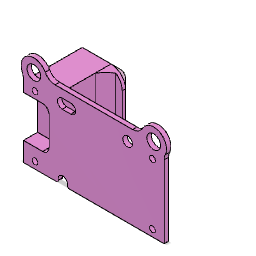
Vindriktning-Cubecell-Mount (Autodesk Fusion 360 design; units mm, degrees)
Autodesk Fusion 360 part; units mm, degrees
sketch "Sketch1" plane through (0, 0, 0) normal (0, 0, 1) x (1, 0, 0)
  line L0 (18.75, 13) -> (-18.75, 13)
  line L1 (-18.75, 13) -> (-18.75, -13)
  line L2 (-18.75, -13) -> (18.75, -13)
  line L3 (18.75, -13) -> (18.75, 13)
  line L4 (18.75, 13) -> (-18.75, -13) construction
  line L5 (-18.75, 13) -> (18.75, -13) construction
  circle A0 centre (18.75, 13) radius 2
  circle A1 centre (-18.75, 13) radius 2
  circle A2 centre (-18.75, 13) radius 4
  circle A3 centre (18.75, 13) radius 4
  line L6 (-18.75, 13) -> (-22, 13)
  line L7 (-22, 13) -> (-22, -13)
  line L8 (-22, -13) -> (-18.75, -13)
  line L9 (-18.75, -13) -> (-18.75, 13)
  line L10 (0, 6) -> (0, -5)
  line L11 (18.75, -13) -> (18.75, 13)
  line L12 (18.75, 13) -> (22, 13)
  line L13 (22, -13) -> (18.75, -13)
  line L14 (22, 13) -> (22, -13)
  line L15 (-22, -6) -> (-14, -6)
  line L16 (-14, -6) -> (-14, 6)
  line L17 (-14, 6) -> (-22, 6)
  line L18 (-22, 6) -> (-22, -6)
  circle A4 centre (-18.75, 13) radius 2.15
  circle A5 centre (18.75, 13) radius 2.15
  dimension "d1" = 37.5
  dimension "d2" = 26
  dimension "d3" = 4
  dimension "d4" = 4
  dimension "d5" = 2
  dimension "d6" = 2
  dimension "d7" = 8
  dimension "d8" = 0.15
  dimension "d9" = 0.15
  constraint horizontal L0
  constraint perpendicular L0 L1
  constraint parallel L0 L2
  constraint parallel L1 L3
  constraint coincident L4 origin
  constraint coincident L5 origin
  constraint coincident L0.start L3.end
  constraint coincident L0.end L1.start
  constraint horizontal L6
  constraint vertical L7
  constraint horizontal L8
  constraint vertical L9
  constraint vertical L10
  constraint symmetric L0.end L10 L0.start
  constraint symmetric L6.end L10 L12.end
  constraint symmetric L7.end L10 L13.start
  constraint symmetric L1.end L10 L2.end
  constraint horizontal L15
  constraint vertical L16
  constraint horizontal L17
  constraint vertical L18
  constraint coincident L7 L15.start
  measures "d1" distance of L1.end L2.end
  measures "d2" distance of L0.end L1.end
  measures "d3" diameter of A0
  measures "d4" diameter of A1
  measures "d5" distance of A1
  measures "d6" distance of A0
  measures "d7" distance of L15.start L15.end
extrude "Extrude1" add sketch "Sketch1" along normal blind 1.4 contours L0 L1 A2 L9 A4 | L0 A2 L6 L7 A4 | L0 L1 L2 L3 A2 A3 L9 L11 L15 L16 L17 | L0 A3 L12 L14 A5 | L0 L3 A3 L11 A5 | L1 A2 L6 L7 L9 A4 | L1 A2 L7 L9 L17 | L3 A3 L11 L13 L14 | L3 A3 L11 L12 L14 A5 | L1 L7 L8 L9 L15
fillet "Fillet1" radius 3.5 2 edges at (-14.75, 13, 0.7) (14.75, 13, 0.7)
fillet "Fillet2" radius 3.5 2 edges at (22, 10.6682, 0.7) (-22, 10.6682, 0.7)
sketch "Sketch2" plane through (0, 0, 1.4) normal (0, 0, 1) x (1, 0, 0)
  circle A0 centre (18.75, 13) radius 2.15
  circle A1 centre (-18.75, 13) radius 2.15
  line L0 (-22, -6) -> (-22, -13)
  line L1 (-22, -13) -> (22, -13)
  line L2 (22, -13) -> (22, 9.7308)
  arc A2 (22.35, 11.2564) -> (22, 9.7308) centre (25.5, 9.7308) ccw
  arc A3 (22.35, 11.2564) -> (15.2123, 14.8667) centre (18.75, 13) ccw
  arc A4 (12.1168, 13) -> (15.2123, 14.8667) centre (12.1168, 16.5) ccw
  line L3 (12.1168, 13) -> (-12.1168, 13)
  arc A5 (-15.2123, 14.8667) -> (-12.1168, 13) centre (-12.1168, 16.5) ccw
  arc A6 (-15.2123, 14.8667) -> (-22.35, 11.2564) centre (-18.75, 13) ccw
  arc A7 (-22, 9.7308) -> (-22.35, 11.2564) centre (-25.5, 9.7308) ccw
  line L4 (-22, 9.7308) -> (-22, 6)
  line L5 (-22, 6) -> (-14, 6)
  line L6 (-14, 6) -> (-14, -6)
  line L7 (-14, -6) -> (-22, -6)
  line L8 (20.375, 10.1157) -> (-20.375, 10.1157)
  line L9 (-20.375, 10.1157) -> (-20.375, -12.8843)
  line L10 (-20.375, -12.8843) -> (20.375, -12.8843)
  line L11 (20.375, -12.8843) -> (20.375, 10.1157)
  line L12 (20.375, 10.1157) -> (-20.375, -12.8843) construction
  line L13 (-20.375, 10.1157) -> (20.375, -12.8843) construction
  point P0 (0, -1.3843)
  point P1 (18.375, 8.1157)
  point P2 (-18.375, 8.1157)
  point P3 (-18.375, -10.8843)
  point P4 (18.375, -10.8843)
  dimension "d16" = 40.75
  dimension "d17" = 23
  dimension "d18" = 2
  dimension "d19" = 2
  dimension "d20" = 2
  dimension "d21" = 2
  dimension "d22" = 2
  dimension "d23" = 2
  dimension "d24" = 2
  dimension "d25" = 2
  constraint horizontal L8
  constraint perpendicular L8 L9
  constraint parallel L8 L10
  constraint parallel L9 L11
  constraint coincident L12 P0
  constraint coincident L13 P0
  measures "d16" distance of L9.end L10.end
  measures "d17" distance of L8.end L9.end
  measures "d18" distance of L8 P1
  measures "d19" distance of L11 P1
  measures "d20" distance of L9 P3
  measures "d21" distance of L9 P2
  measures "d22" distance of L8 P2
  measures "d23" distance of L10 P3
  measures "d24" distance of L11 P4
  measures "d25" distance of L10 P4
hole "Hole1" at (-18.375, 8.1157, 1.4) at (-18.375, -10.8843, 1.4) at (18.375, -10.8843, 1.4) at (18.375, 8.1157, 1.4) direction (0, 0, -1) diameter 1.8 end up to surface (1.4 mm away)
extrude "Extrude2" cut 1 faces at (-16.6667, -6, 0.9333) along direction (0, -1, 0) blind 1
fillet "Fillet3" radius 2 2 edges at (-14, 6, 0.7) (-14, -7, 0.7)
sketch "Sketch3" plane through (0, 0, 0) normal (0, 0, -1) x (-1, 0, 0)
  line L0 (22, -7) -> (16, -7)
  arc A0 (14, -5) -> (16, -7) centre (16, -5) ccw
  line L1 (14, -5) -> (14, 4)
  arc A1 (16, 6) -> (14, 4) centre (16, 4) ccw
  line L2 (16, 6) -> (22, 6)
  line L3 (22, 6) -> (22, 9.7308)
  arc A2 (22.35, 11.2564) -> (22, 9.7308) centre (25.5, 9.7308) ccw
  arc A3 (22.35, 11.2564) -> (15.2123, 14.8667) centre (18.75, 13) ccw
  arc A4 (12.1168, 13) -> (15.2123, 14.8667) centre (12.1168, 16.5) ccw
  line L4 (12.1168, 13) -> (-12.1168, 13)
  arc A5 (-15.2123, 14.8667) -> (-12.1168, 13) centre (-12.1168, 16.5) ccw
  arc A6 (-15.2123, 14.8667) -> (-22.35, 11.2564) centre (-18.75, 13) ccw
  arc A7 (-22, 9.7308) -> (-22.35, 11.2564) centre (-25.5, 9.7308) ccw
  line L5 (-22, 9.7308) -> (-22, -13)
  line L6 (-22, -13) -> (22, -13)
  line L7 (22, -13) -> (22, -7)
  circle A8 centre (18.75, 13) radius 2.15
  circle A9 centre (-18.75, 13) radius 2.15
  circle A10 centre (-18.375, 8.1157) radius 0.9
  circle A11 centre (18.375, -10.8843) radius 0.9
  circle A12 centre (18.375, 8.1157) radius 0.9
  circle A13 centre (-18.375, -10.8843) radius 0.9
  line L8 (22, -13) -> (13, -13)
  line L9 (13, -13) -> (13, 9)
  line L10 (13, 9) -> (22, 9)
  line L11 (22, 9) -> (22, -13)
  constraint horizontal L8
  constraint vertical L9
  constraint horizontal L10
  constraint vertical L11
  constraint coincident L6.end L7.start
extrude "Extrude3" add sketch "Sketch3" along normal blind 20 contours L0 A0 L1 A1 L2 L3 L6 L7 A12 L8 L9 L10 L11 | A12 L10 | A11 picked at (18.3114, 7.9506)
sketch "Sketch4" plane through (0, 0, -20) normal (0, 0, -1) x (-1, 0, 0)
  line L0 (22, -7) -> (16, -7)
  arc A0 (14, -5) -> (16, -7) centre (16, -5) ccw
  line L1 (14, -5) -> (14, 4)
  arc A1 (16, 6) -> (14, 4) centre (16, 4) ccw
  line L2 (16, 6) -> (22, 6)
  line L3 (22, 6) -> (22, 9)
  line L4 (22, 9) -> (13, 9)
  line L5 (13, 9) -> (13, -13)
  line L6 (13, -13) -> (22, -13)
  line L7 (22, -13) -> (22, -7)
  line L8 (22, 6) -> (22, -6)
  line L9 (22, 13) -> (22, -13)
  circle A2 centre (-18.375, -10.8843) radius 0.9
  line L10 (13, -13) -> (13, 9)
  line L11 (13, 9) -> (18.2077, 9)
  arc A3 (18.5423, 9) -> (18.2077, 9) centre (18.375, 8.1157) ccw
  line L12 (18.5423, 9) -> (22, 9)
  line L13 (22, 9) -> (22, 9.7308)
  arc A4 (22.35, 11.2564) -> (22, 9.7308) centre (25.5, 9.7308) ccw
  arc A5 (22.35, 11.2564) -> (15.2123, 14.8667) centre (18.75, 13) ccw
  arc A6 (12.1168, 13) -> (15.2123, 14.8667) centre (12.1168, 16.5) ccw
  line L14 (12.1168, 13) -> (-12.1168, 13)
  arc A7 (-15.2123, 14.8667) -> (-12.1168, 13) centre (-12.1168, 16.5) ccw
  arc A8 (-15.2123, 14.8667) -> (-22.35, 11.2564) centre (-18.75, 13) ccw
  arc A9 (-22, 9.7308) -> (-22.35, 11.2564) centre (-25.5, 9.7308) ccw
  line L15 (-22, 9.7308) -> (-22, -13)
  line L16 (-22, -13) -> (13, -13)
  circle A10 centre (-18.375, 8.1157) radius 0.9
  circle A11 centre (-18.75, 13) radius 2.15
  circle A12 centre (18.75, 13) radius 2.15
extrude "Extrude4" add sketch "Sketch4" against normal blind 17 contours L0 A0 L1 A1 L2 L8 L9
sketch "Sketch5" plane through (-13, 0, 0) normal (1, 0, 0) x (0, 0, -1)
  line L0 (0, 9) -> (0, -13)
  line L1 (0, -13) -> (20, -13)
  line L2 (20, -13) -> (20, 9)
  line L3 (20, 9) -> (0, 9)
  line L4 (20, 9) -> (16, 9)
  line L5 (16, 9) -> (16, -13)
  line L6 (16, -13) -> (20, -13)
  line L7 (20, -13) -> (20, 9)
  dimension "d37" = 4
  constraint horizontal L4
  constraint vertical L5
  constraint horizontal L6
  constraint vertical L7
  constraint coincident L2.end L3.start
  measures "d37" distance of L2.end L4.end
extrude "Extrude5" add sketch "Sketch5" along normal blind 4.5 contours L1 L2 L3 L4 L5 L6 L7
fillet "Fillet4" radius 4.5 2 edges at (-8.5, 9, -18) (-8.5, -13, -18)
chamfer "Chamfer1" distance 3 angle 45 5 edges at (-8.5, -2, -20) (-9.818, 7.682, -20) (-17.5, 9, -20) (-17.5, -13, -20) (-9.818, -11.682, -20)
sketch "Sketch6" plane through (0, 0, 1.4) normal (0, 0, 1) x (1, 0, 0)
  line L0 (-14, 4) -> (-14, -5)
  arc A0 (-16, -7) -> (-14, -5) centre (-16, -5) ccw
  line L1 (-16, -7) -> (-22, -7)
  line L2 (-22, -7) -> (-22, -13)
  line L3 (-22, -13) -> (22, -13)
  line L4 (22, -13) -> (22, 9.7308)
  arc A1 (22.35, 11.2564) -> (22, 9.7308) centre (25.5, 9.7308) ccw
  arc A2 (22.35, 11.2564) -> (15.2123, 14.8667) centre (18.75, 13) ccw
  arc A3 (12.1168, 13) -> (15.2123, 14.8667) centre (12.1168, 16.5) ccw
  line L5 (12.1168, 13) -> (-12.1168, 13)
  arc A4 (-15.2123, 14.8667) -> (-12.1168, 13) centre (-12.1168, 16.5) ccw
  arc A5 (-15.2123, 14.8667) -> (-22.35, 11.2564) centre (-18.75, 13) ccw
  arc A6 (-22, 9.7308) -> (-22.35, 11.2564) centre (-25.5, 9.7308) ccw
  line L6 (-22, 9.7308) -> (-22, 6)
  line L7 (-22, 6) -> (-16, 6)
  arc A7 (-14, 4) -> (-16, 6) centre (-16, 4) ccw
  circle A8 centre (-18.75, 13) radius 2.15
  circle A9 centre (18.75, 13) radius 2.15
  circle A10 centre (18.375, 8.1157) radius 0.9
  circle A11 centre (-18.375, -10.8843) radius 0.9
  circle A12 centre (-18.375, 8.1157) radius 0.9
  circle A13 centre (18.375, -10.8843) radius 0.9
  circle A14 centre (10.575, 9) radius 1.5
  line L8 (18.75, 13) -> (-18.75, 13)
  line L9 (-9.875, 7.5) -> (-7.175, 7.5)
  arc A15 (-7.175, 7.5) -> (-7.175, 10.5) centre (-7.175, 9) ccw
  line L10 (-7.175, 10.5) -> (-9.875, 10.5)
  arc A16 (-9.875, 10.5) -> (-9.875, 7.5) centre (-9.875, 9) ccw
  line L11 (-9.875, 9) -> (-7.175, 9) construction
  circle A17 centre (-9.7, -12) radius 1.5
  line L12 (-18.75, -13) -> (18.75, -13)
  line L13 (-22, 13) -> (-22, -13)
  dimension "d43" = 3
  dimension "d44" = 7.8
  dimension "d45" = 4
  dimension "d46" = 3
  dimension "d47" = 4
  dimension "d48" = 17.75
  dimension "d49" = 3
  dimension "d50" = 1
  dimension "d51" = 12.3
  constraint tangent L9 A15
  constraint tangent A15 L10
  constraint parallel L9 L10
  constraint tangent L10 A16
  constraint tangent L9 A16
  constraint parallel L8 L11
  measures "d43" diameter of A14
  measures "d44" horizontal distance of A10.centre A14.centre
  measures "d45" distance of A14.centre L8
  measures "d46" diameter of A15
  measures "d47" distance of L8 A15.centre
  measures "d48" distance of A14.centre A15.centre
  measures "d49" diameter of A17
  measures "d50" distance of A17.centre L12
  measures "d51" distance of A17.centre L13
extrude "Extrude6" cut sketch "Sketch6" against normal up to surface (1.4 mm away) contours L3 A17 L12 | A14 | L9 A15 L10 A16 picked at (-9.2869, -11.8591)
fillet "Fillet5" radius 0.5 2 edges at (-10.818, -13, 0.7) (-8.582, -13, 0.7)
chamfer "Chamfer2" distance 4 distance2 2.5 1 edges at (-13, -2, -16) measured on face at (-13, -5.6667, -10.6667)
equation "d35 = -21.00 mm + 4 mm"
